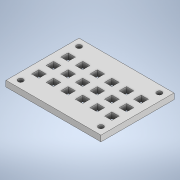
# Autodesk Inventor part: floor_plan
Saved by Autodesk Inventor 2022 (Build 260153000, 153)
## iProperties
Created: 2024-03-25
Part Number: floor_plan
Material: Generic
Document SubType Name: Modeling
Designer: subin
Density: 1 g/cm^3
Appearance: Default
Author: subin
Autodesk Inventor part; units mm, degrees
ref_plane "YZ Plane" through (0, 0, 0) normal (1, 0, 0) x (0, 1, 0)
ref_plane "XZ Plane" through (0, 0, 0) normal (0, 1, 0) x (-1, 0, 0)
ref_plane "XY Plane" through (0, 0, 0) normal (0, 0, 1) x (1, 0, 0)
sketch "Sketch1" plane through (0, 0, 0) normal (0, 1, 0) x (-1, 0, 0)
  line L0 (0, 0) -> (130, 0)
  line L1 (130, 0) -> (130, -100)
  line L2 (130, -100) -> (0, -100)
  line L3 (0, -100) -> (0, 0)
  dimension "d0" = 130
  dimension "d1" = 100
  constraints: 8 end point, 2 parallel, 1 horizontal, 1 perpendicular
  measures "d0" distance of L1.end L2.end
  measures "d1" distance of L2.end L0.start
extrude "Extrusion1" add sketch "Sketch1" along normal blind 8
sketch "Sketch3" plane through (0, 8, 0) normal (0, 1, 0) x (1, 0, 0)
  line L0 (-120, 5) -> (-110, 5)
  line L1 (-110, 5) -> (-110, 15)
  line L2 (-110, 15) -> (-120, 15)
  line L3 (-120, 15) -> (-120, 5)
  line L4 (-130, 100) -> (-130, 0) projected
  line L5 (-130, 0) -> (0, 0) projected
  line L6 (-105, 0) -> (-105, 100)
  line L7 (0, 100) -> (-130, 100) projected
  line L8 (-130, 20) -> (-105, 20)
  line L9 (-120, 35) -> (-110, 35)
  line L10 (-110, 35) -> (-110, 25)
  line L11 (-110, 25) -> (-120, 25)
  line L12 (-120, 25) -> (-120, 35)
  line L13 (-130, 40) -> (-105, 40)
  line L14 (-120, 75) -> (-110, 75)
  line L15 (-110, 75) -> (-110, 65)
  line L16 (-110, 65) -> (-120, 65)
  line L17 (-120, 65) -> (-120, 75)
  line L18 (-120, 45) -> (-110, 45)
  line L19 (-110, 45) -> (-110, 55)
  line L20 (-110, 55) -> (-120, 55)
  line L21 (-120, 55) -> (-120, 45)
  line L22 (-130, 80) -> (-105, 80)
  line L23 (-120, 155) -> (-110, 155)
  line L24 (-110, 155) -> (-110, 145)
  line L25 (-110, 145) -> (-120, 145)
  line L26 (-120, 145) -> (-120, 155)
  line L27 (-130, 100) -> (0, 100)
  line L28 (-120, 125) -> (-110, 125)
  line L29 (-110, 125) -> (-110, 135)
  line L30 (-110, 135) -> (-120, 135)
  line L31 (-120, 135) -> (-120, 125)
  line L32 (-110, 95) -> (-120, 95)
  line L33 (-120, 95) -> (-120, 85)
  line L34 (-110, 105) -> (-120, 105)
  line L35 (-120, 85) -> (-110, 85)
  line L36 (-110, 85) -> (-110, 95)
  line L37 (-120, 105) -> (-120, 115)
  line L38 (-120, 115) -> (-110, 115)
  line L39 (-110, 115) -> (-110, 105)
  line L40 (-90, 5) -> (-100, 5)
  line L41 (-100, 5) -> (-100, 15)
  line L42 (-100, 15) -> (-90, 15)
  line L43 (-90, 15) -> (-90, 5)
  line L44 (-90, 35) -> (-100, 35)
  line L45 (-100, 35) -> (-100, 25)
  line L46 (-100, 25) -> (-90, 25)
  line L47 (-90, 25) -> (-90, 35)
  line L48 (-100, 65) -> (-90, 65)
  line L49 (-90, 65) -> (-90, 75)
  line L50 (-100, 55) -> (-90, 55)
  line L51 (-90, 75) -> (-100, 75)
  line L52 (-100, 75) -> (-100, 65)
  line L53 (-90, 55) -> (-90, 45)
  line L54 (-90, 45) -> (-100, 45)
  line L55 (-100, 45) -> (-100, 55)
  line L56 (-100, 105) -> (-90, 105)
  line L57 (-90, 105) -> (-90, 115)
  line L58 (-100, 115) -> (-100, 105)
  line L59 (-90, 115) -> (-100, 115)
  line L60 (-90, 125) -> (-100, 125)
  line L61 (-100, 125) -> (-100, 135)
  line L62 (-100, 135) -> (-90, 135)
  line L63 (-90, 135) -> (-90, 125)
  line L64 (-90, 155) -> (-100, 155)
  line L65 (-100, 155) -> (-100, 145)
  line L66 (-100, 145) -> (-90, 145)
  line L67 (-90, 145) -> (-90, 155)
  line L68 (-90, 95) -> (-90, 85)
  line L69 (-90, 85) -> (-100, 85)
  line L70 (-100, 85) -> (-100, 95)
  line L71 (-100, 95) -> (-90, 95)
  line L72 (-85, 0) -> (-85, 100)
  line L73 (-50, 5) -> (-60, 5)
  line L74 (-60, 5) -> (-60, 15)
  line L75 (-60, 15) -> (-50, 15)
  line L76 (-50, 15) -> (-50, 5)
  line L77 (-50, 35) -> (-60, 35)
  line L78 (-60, 35) -> (-60, 25)
  line L79 (-60, 25) -> (-50, 25)
  line L80 (-50, 25) -> (-50, 35)
  line L81 (-60, 65) -> (-50, 65)
  line L82 (-50, 65) -> (-50, 75)
  line L83 (-60, 55) -> (-50, 55)
  line L84 (-50, 75) -> (-60, 75)
  line L85 (-60, 75) -> (-60, 65)
  line L86 (-50, 55) -> (-50, 45)
  line L87 (-50, 45) -> (-60, 45)
  line L88 (-60, 45) -> (-60, 55)
  line L89 (-60, 105) -> (-50, 105)
  line L90 (-50, 105) -> (-50, 115)
  line L91 (-60, 115) -> (-60, 105)
  line L92 (-50, 115) -> (-60, 115)
  line L93 (-50, 125) -> (-60, 125)
  line L94 (-60, 125) -> (-60, 135)
  line L95 (-60, 135) -> (-50, 135)
  line L96 (-50, 135) -> (-50, 125)
  line L97 (-50, 155) -> (-60, 155)
  line L98 (-60, 155) -> (-60, 145)
  line L99 (-60, 145) -> (-50, 145)
  line L100 (-50, 145) -> (-50, 155)
  line L101 (-50, 95) -> (-50, 85)
  line L102 (-50, 85) -> (-60, 85)
  line L103 (-60, 85) -> (-60, 95)
  line L104 (-60, 95) -> (-50, 95)
  line L105 (-80, 125) -> (-70, 125)
  line L106 (-70, 125) -> (-70, 135)
  line L107 (-80, 135) -> (-80, 125)
  line L108 (-70, 135) -> (-80, 135)
  line L109 (-70, 145) -> (-80, 145)
  line L110 (-80, 155) -> (-70, 155)
  line L111 (-80, 145) -> (-80, 155)
  line L112 (-70, 155) -> (-70, 145)
  line L113 (-70, 15) -> (-80, 15)
  line L114 (-80, 15) -> (-80, 5)
  line L115 (-80, 5) -> (-70, 5)
  line L116 (-70, 5) -> (-70, 15)
  line L117 (-80, 45) -> (-70, 45)
  line L118 (-80, 35) -> (-70, 35)
  line L119 (-70, 25) -> (-80, 25)
  line L120 (-80, 25) -> (-80, 35)
  line L121 (-70, 35) -> (-70, 25)
  line L122 (-70, 45) -> (-70, 55)
  line L123 (-80, 55) -> (-80, 45)
  line L124 (-70, 65) -> (-80, 65)
  line L125 (-70, 75) -> (-70, 65)
  line L126 (-80, 65) -> (-80, 75)
  line L127 (-80, 75) -> (-70, 75)
  line L128 (-70, 55) -> (-80, 55)
  line L129 (-80, 85) -> (-70, 85)
  line L130 (-70, 85) -> (-70, 95)
  line L131 (-80, 95) -> (-80, 85)
  line L132 (-70, 95) -> (-80, 95)
  line L133 (-70, 105) -> (-80, 105)
  line L134 (-80, 115) -> (-70, 115)
  line L135 (-80, 105) -> (-80, 115)
  line L136 (-70, 115) -> (-70, 105)
  line L137 (-45, 0) -> (-45, 100)
  line L138 (-10, 125) -> (-20, 125)
  line L139 (-20, 125) -> (-20, 135)
  line L140 (-10, 135) -> (-10, 125)
  line L141 (-20, 135) -> (-10, 135)
  line L142 (-20, 145) -> (-10, 145)
  line L143 (-20, 155) -> (-20, 145)
  line L144 (-10, 155) -> (-20, 155)
  line L145 (-10, 145) -> (-10, 155)
  line L146 (-40, 5) -> (-30, 5)
  line L147 (-30, 5) -> (-30, 15)
  line L148 (-30, 15) -> (-40, 15)
  line L149 (-40, 15) -> (-40, 5)
  line L150 (-40, 65) -> (-40, 75)
  line L151 (-40, 35) -> (-30, 35)
  line L152 (-30, 35) -> (-30, 25)
  line L153 (-30, 25) -> (-40, 25)
  line L154 (-40, 25) -> (-40, 35)
  line L155 (-30, 65) -> (-40, 65)
  line L156 (-40, 75) -> (-30, 75)
  line L157 (-30, 75) -> (-30, 65)
  line L158 (-30, 55) -> (-40, 55)
  line L159 (-40, 55) -> (-40, 45)
  line L160 (-40, 45) -> (-30, 45)
  line L161 (-30, 45) -> (-30, 55)
  line L162 (-30, 125) -> (-30, 135)
  line L163 (-30, 155) -> (-30, 145)
  line L164 (-40, 125) -> (-30, 125)
  line L165 (-40, 135) -> (-40, 125)
  line L166 (-30, 135) -> (-40, 135)
  line L167 (-30, 145) -> (-40, 145)
  line L168 (-40, 145) -> (-40, 155)
  line L169 (-40, 155) -> (-30, 155)
  line L170 (-30, 105) -> (-40, 105)
  line L171 (-40, 105) -> (-40, 115)
  line L172 (-30, 115) -> (-30, 105)
  line L173 (-40, 115) -> (-30, 115)
  line L174 (-40, 95) -> (-40, 85)
  line L175 (-40, 85) -> (-30, 85)
  line L176 (-30, 85) -> (-30, 95)
  line L177 (-30, 95) -> (-40, 95)
  line L178 (-10, 115) -> (-20, 115)
  line L179 (-20, 115) -> (-20, 105)
  line L180 (-10, 105) -> (-10, 115)
  line L181 (-20, 105) -> (-10, 105)
  line L182 (-20, 95) -> (-10, 95)
  line L183 (-20, 85) -> (-20, 95)
  line L184 (-10, 85) -> (-20, 85)
  line L185 (-10, 95) -> (-10, 85)
  line L186 (-10, 75) -> (-20, 75)
  line L187 (-10, 65) -> (-10, 75)
  line L188 (-20, 65) -> (-10, 65)
  line L189 (-20, 75) -> (-20, 65)
  line L190 (-20, 15) -> (-10, 15)
  line L191 (-10, 15) -> (-10, 5)
  line L192 (-20, 5) -> (-20, 15)
  line L193 (-10, 5) -> (-20, 5)
  line L194 (-10, 45) -> (-20, 45)
  line L195 (-10, 35) -> (-20, 35)
  line L196 (-10, 25) -> (-10, 35)
  line L197 (-20, 25) -> (-10, 25)
  line L198 (-20, 55) -> (-10, 55)
  line L199 (-20, 45) -> (-20, 55)
  line L200 (-20, 35) -> (-20, 25)
  line L201 (-10, 55) -> (-10, 45)
  point P0 (-65, 20)
  point P1 (-65, 40)
  point P2 (-65, 80)
  point P3 (-25, 20)
  point P4 (-25, 40)
  point P5 (-25, 80)
  dimension "d21" = 10
  dimension "d22" = 10
  dimension "d23" = 10
  dimension "d24" = 5
  dimension "d25" = 5
  dimension "d26" = 5
  dimension "d27" = 5
  dimension "d28" = 5
  dimension "d29" = 5
  dimension "d30" = 5
  dimension "d40" = 5
  constraints: 398 end point, 194 symmetric about line, 12 point on line, 6 perpendicular, 2 parallel, 1 horizontal, 1 vertical
  measures "d21" distance of L2.end L1.end
  measures "d22" distance of L1.end L0.end
  measures "d23" distance between parallel lines of L4 L3
  measures "d24" distance between parallel lines of L5 L0
  measures "d25" distance between parallel lines of L8 L2
  measures "d26" distance between parallel lines of L13 L9
  measures "d27" distance between parallel lines of L22 L14
  measures "d28" distance between parallel lines of L6 L24
  measures "d29" distance between parallel lines of L72 L49
  measures "d30" distance between parallel lines of L137 L100
  measures "d40" distance between parallel lines of L7 L32
sketch "Sketch4" plane through (0, 8, 0) normal (0, 1, 0) x (1, 0, 0)
  circle A0 centre (-120, 10) radius 3.5
  line L0 (-130, 0) -> (0, 0) projected
  line L1 (-130, 100) -> (-130, 0) projected
  line L2 (-65, 0) -> (-65, 170)
  line L3 (-130, 100) -> (-130, 0) projected
  line L4 (-130, 50) -> (0, 50)
  circle A1 centre (-10, 10) radius 3.5
  circle A2 centre (-120, 90) radius 3.5
  line L5 (-130, 100) -> (0, 100)
  circle A3 centre (-10, 90) radius 3.5
  point P0 (0, 100)
  dimension "d35" = 7
  dimension "d36" = 10
  dimension "d37" = 10
  constraints: 4 centre point, 4 end point, 4 symmetric about line, 2 midpoint, 1 horizontal, 1 vertical, 6 other
  measures "d35" diameter of A0
  measures "d36" distance from line of L0 A0.centre
  measures "d37" distance from line of L1 A0.centre
extrude "Extrusion5" cut sketch "Sketch4" against normal blind 20 contours A0 | A1 | A2 | A3
extrude "Extrusion6" cut sketch "Sketch3" against normal blind 20 contours L9 L10 L11 L12 | L14 L15 L16 L17 | L21 L20 L19 L18 | L47 L46 L45 L44 | L52 L51 L49 L48 | L50 L53 L54 L55 | L80 L79 L78 L77 | L85 L84 L82 L81 | L83 L86 L87 L88 | L123 L128 L122 L117 | L118 L121 L119 L120 | L124 L126 L127 L125 | L150 L156 L157 L155 | L151 L152 L153 L154 | L161 L160 L159 L158 | L187 L188 L189 L186 | L194 L199 L198 L201 | L196 L197 L200 L195
body "Solid1"
